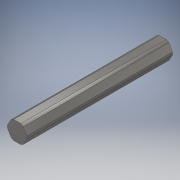
# Autodesk Inventor part: drive_shaft
Saved by Autodesk Inventor 2019.3 (Build 233278000, 278)
## iProperties
Created: 2019-04-09
Part Number: drive_shaft
Material: Steel, Alloy
Document SubType Name: Modeling
Designer: Connor
Density: 7.73 g/cm^3
Appearance: Semi-Polished
Author: Connor
Autodesk Inventor part; units mm, degrees
ref_plane "YZ Plane" through (0, 0, 0) normal (1, 0, 0) x (0, 1, 0)
ref_plane "XZ Plane" through (0, 0, 0) normal (0, 1, 0) x (-1, 0, 0)
ref_plane "XY Plane" through (0, 0, 0) normal (0, 0, 1) x (1, 0, 0)
sketch "Sketch1" plane through (0, 0, 0) normal (0, 0, 1) x (1, 0, 0)
  line L0 (2.7496, 4.7625) -> (3.1778, 4.0208)
  line L1 (5.4993, 0) -> (5.071, -0.7417)
  line L2 (2.7496, -4.7625) -> (1.8932, -4.7625)
  line L3 (-2.7496, -4.7625) -> (-3.1778, -4.0208)
  line L4 (-5.4993, 0) -> (-5.071, 0.7417)
  line L5 (-2.7496, 4.7625) -> (-1.8932, 4.7625)
  arc A0 (-3.1778, -4.0208) -> (-1.8932, -4.7625) centre (0, 0) ccw
  line L6 (-3.1778, 4.0208) -> (-2.7496, 4.7625)
  line L7 (1.8932, 4.7625) -> (2.7496, 4.7625)
  line L8 (5.071, 0.7417) -> (5.4993, 0)
  line L9 (5.071, -0.7417) -> (3.1778, -4.0208)
  line L10 (-1.8932, -4.7625) -> (-2.7496, -4.7625)
  line L11 (-3.1778, -4.0208) -> (-5.071, -0.7417)
  arc A1 (-5.071, -0.7417) -> (-3.1778, -4.0208) centre (0, 0) ccw
  arc A2 (-5.071, 0.7417) -> (-5.071, -0.7417) centre (0, 0) ccw
  arc A3 (-3.1778, 4.0208) -> (-5.071, 0.7417) centre (0, 0) ccw
  arc A4 (-1.8932, 4.7625) -> (-3.1778, 4.0208) centre (0, 0) ccw
  arc A5 (5.071, 0.7417) -> (3.1778, 4.0208) centre (0, 0) ccw
  arc A6 (5.071, -0.7417) -> (5.071, 0.7417) centre (0, 0) ccw
  arc A7 (-1.8932, -4.7625) -> (1.8932, -4.7625) centre (0, 0) ccw
  arc A8 (1.8932, -4.7625) -> (3.1778, -4.0208) centre (0, 0) ccw
  arc A9 (3.1778, -4.0208) -> (5.071, -0.7417) centre (0, 0) ccw
  arc A10 (3.1778, 4.0208) -> (1.8932, 4.7625) centre (0, 0) ccw
  arc A11 (1.8932, 4.7625) -> (-1.8932, 4.7625) centre (0, 0) ccw
  line L12 (-5.071, 0.7417) -> (-3.1778, 4.0208)
  line L13 (-5.071, -0.7417) -> (-5.4993, 0)
  line L14 (1.8932, -4.7625) -> (-1.8932, -4.7625)
  line L15 (3.1778, -4.0208) -> (2.7496, -4.7625)
  line L16 (3.1778, 4.0208) -> (5.071, 0.7417)
  line L17 (-1.8932, 4.7625) -> (1.8932, 4.7625)
  dimension "d0" = 9.525
  dimension "d1" = 10.25
  constraints: 42 point on circle, 36 end point, 12 centre point, 2 coincident, 13 other
  measures "d0" distance between parallel lines of L2 L5
  measures "d1" diameter of A0
extrude "Extrusion1" add sketch "Sketch1" along normal blind 76.2 contours L16 A6 L9 A8 L14 A0 L11 A2 L12 A4 L17 A10
body "Solid1"
